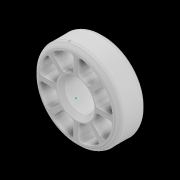
# Autodesk Inventor part: ToroidalCore
Saved by Autodesk Inventor 2020.4 (Build 244396010, 396A)
## iProperties
Created: 2022-09-12
Part Number: ToroidalCore
Material: Generic
Document SubType Name: Modeling
Designer: Val
Density: 1 g/cm^3
Appearance: Default
Author: Val
Autodesk Inventor part; units mm, degrees
ref_plane "YZ Plane" through (0, 0, 0) normal (1, 0, 0) x (0, 1, 0)
ref_plane "XZ Plane" through (0, 0, 0) normal (0, 1, 0) x (-1, 0, 0)
ref_plane "XY Plane" through (0, 0, 0) normal (0, 0, 1) x (1, 0, 0)
sketch "Sketch1" plane through (0, 0, 0) normal (0, 0, 1) x (1, 0, 0)
  circle A0 centre (0, 0) radius 91.25
  circle A1 centre (0, 0) radius 31.75
  dimension "d0" = 182.5
  dimension "d1" = 63.5
  constraints: 2 centre point, 2 coincident
  measures "d0" diameter of A0
  measures "d1" diameter of A1
extrude "Extrusion1" add sketch "Sketch1" along normal blind 59.945
chamfer "Chamfer1" distance 8.4582 angle 45 4 edges at (-91.25, 0, 59.945) (-31.75, 0, 59.945) (-91.25, 0, 0) (-31.75, 0, 0)
fillet "Fillet1" radius 6.35 4 edges at (-91.25, 0, 51.4868) (-82.7918, 0, 59.945) (-91.25, 0, 8.4582) (-82.7918, 0, 0)
sketch "Sketch2" plane through (0, 0, 59.945) normal (0, 0, 1) x (1, 0, 0)
  point P0 (0, 0)
sketch "Sketch3" plane through (0, 0, 59.945) normal (0, 0, 1) x (1, 0, 0)
  circle A0 centre (0, 0) radius 40.2082 construction
  circle A1 centre (0, 0) radius 80.1615 construction
  line L0 (0, 0) -> (0, -80.1615) construction
  line L1 (0, 0) -> (0, 80.1615) construction
  circle A2 centre (0, 0) radius 80.1615 construction
  line L2 (0, 0) -> (-80.1615, 0) construction
  line L3 (0, 0) -> (80.1615, 0) construction
  line L4 (0, 0) -> (56.6828, -56.6828) construction
  arc A3 (5, -78.0015) -> (51.6198, -58.6909) centre (0, 0) ccw
  arc A4 (5, -41.911) -> (26.1, -33.1711) centre (0, 0) ccw
  line L5 (51.6198, -58.6909) -> (26.1, -33.1711)
  line L6 (5, -78.0015) -> (5, -41.911)
  arc A5 (58.6909, -51.6198) -> (78.0015, -5) centre (0, 0) ccw
  arc A6 (33.1711, -26.1) -> (41.911, -5) centre (0, 0) ccw
  line L7 (58.6909, -51.6198) -> (33.1711, -26.1)
  line L8 (78.0015, -5) -> (41.911, -5)
  arc A7 (-51.6198, -58.6909) -> (-5, -78.0015) centre (0, 0) ccw
  arc A8 (-26.1, -33.1711) -> (-5, -41.911) centre (0, 0) ccw
  line L9 (-51.6198, -58.6909) -> (-26.1, -33.1711)
  line L10 (-5, -78.0015) -> (-5, -41.911)
  arc A9 (-78.0015, -5) -> (-58.6909, -51.6198) centre (0, 0) ccw
  line L11 (-58.6909, -51.6198) -> (-33.1711, -26.1)
  line L12 (-78.0015, -5) -> (-41.911, -5)
  arc A10 (-41.911, -5) -> (-33.1711, -26.1) centre (0, 0) ccw
  arc A11 (51.6198, 58.6909) -> (5, 78.0015) centre (0, 0) ccw
  arc A12 (26.1, 33.1711) -> (5, 41.911) centre (0, 0) ccw
  line L13 (51.6198, 58.6909) -> (26.1, 33.1711)
  line L14 (5, 78.0015) -> (5, 41.911)
  arc A13 (78.0015, 5) -> (58.6909, 51.6198) centre (0, 0) ccw
  line L15 (58.6909, 51.6198) -> (33.1711, 26.1)
  line L16 (78.0015, 5) -> (41.911, 5)
  arc A14 (41.911, 5) -> (33.1711, 26.1) centre (0, 0) ccw
  line L17 (-51.6198, 58.6909) -> (-26.1, 33.1711)
  arc A15 (-5, 78.0015) -> (-51.6198, 58.6909) centre (0, 0) ccw
  line L18 (-5, 78.0015) -> (-5, 41.911)
  arc A16 (-5, 41.911) -> (-26.1, 33.1711) centre (0, 0) ccw
  line L19 (-58.6909, 51.6198) -> (-33.1711, 26.1)
  arc A17 (-58.6909, 51.6198) -> (-78.0015, 5) centre (0, 0) ccw
  line L20 (-78.0015, 5) -> (-41.911, 5)
  arc A18 (-33.1711, 26.1) -> (-41.911, 5) centre (0, 0) ccw
  dimension "d8" = 45
  dimension "d9" = 2
  dimension "d10" = 2
  dimension "d11" = 5
  dimension "d12" = 5
  constraints: 44 point on circle, 42 end point, 28 symmetric about line, 16 centre point, 3 vertical, 2 concentric, 2 horizontal, 1 parallel, 1 vertical alignment, 15 other
  measures "d8" angle of L0 L4
  measures "d10" radial gap between concentric circles of A0 A4
  measures "d11" distance between parallel lines of L4 L5
  measures "d12" distance between parallel lines of L0 L6
extrude "Extrusion2" cut sketch "Sketch3" against normal through all
fillet "Fillet2" radius 6.35 32 edges at (51.6198, -58.6909, 29.9725) (5, -78.0015, 29.9725) (26.1, -33.1711, 29.9725) (5, -41.911, 29.9725) (-5, -78.0015, 29.9725) (-5, -41.911, 29.9725) (-51.6198, -58.6909, 29.9725) (-26.1, -33.1711, 29.9725) (-58.6909, -51.6198, 29.9725) (-33.1711, -26.1, 29.9725) (-41.911, -5, 29.9725) (-78.0015, -5, 29.9725) (-78.0015, 5, 29.9725) (-58.6909, 51.6198, 29.9725) (-33.1711, 26.1, 29.9725) (-41.911, 5, 29.9725) (-26.1, 33.1711, 29.9725) (-51.6198, 58.6909, 29.9725) (-5, 78.0015, 29.9725) (-5, 41.911, 29.9725) (5, 41.911, 29.9725) (5, 78.0015, 29.9725) (51.6198, 58.6909, 29.9725) (26.1, 33.1711, 29.9725) (33.1711, 26.1, 29.9725) (58.6909, 51.6198, 29.9725) (78.0015, 5, 29.9725) (41.911, 5, 29.9725) (41.911, -5, 29.9725) (78.0015, -5, 29.9725) (58.6909, -51.6198, 29.9725) (33.1711, -26.1, 29.9725)
sketch "Sketch4" plane through (0, 0, 0) normal (0, 1, 0) x (-1, 0, 0)
  circle A0 centre (23.1161, 50.047) radius 1.5
  point P0 (0, 0)
  dimension "d16" = 3
  constraints: 1 centre point
  measures "d16" diameter of A0
extrude "Extrusion3" cut sketch "Sketch4" along normal through all
equation "\"d10\" = d9"
equation "\"d12\" = d11"
body "Solid1"
